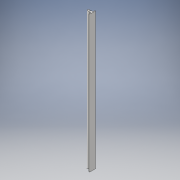
# Autodesk Inventor part: supportedRail_SBR12_750mm
Saved by Autodesk Inventor 2018 (Build 220112000, 112)
## iProperties
Created: 2020-03-10
Part Number: supportedRail_SBR12_750mm
Material: Generic
Document SubType Name: Modeling
Designer: natha
Density: 1 g/cm^3
Appearance: Default
Author: natha
Autodesk Inventor part; units mm, degrees
ref_plane "YZ Plane" through (0, 0, 0) normal (1, 0, 0) x (0, 1, 0)
ref_plane "XZ Plane" through (0, 0, 0) normal (0, 1, 0) x (-1, 0, 0)
ref_plane "XY Plane" through (0, 0, 0) normal (0, 0, 1) x (1, 0, 0)
sketch "Sketch1" plane through (0, 0, 0) normal (0, 1, 0) x (-1, 0, 0)
  line L0 (-22.5, -6) -> (-22.5, 6)
  line L1 (-10.5, -6) -> (-5.8469, -1.3469)
  line L2 (-10.5, -6) -> (-3.9195, -6) construction
  line L3 (-10.5, 6) -> (-5.8469, 1.3469)
  arc A0 (-5.8469, -1.3469) -> (-5.8469, 1.3469) centre (-0.0057, 0) ccw
  line L4 (-22.5, 16) -> (-22.5, -16)
  line L5 (-22.5, -16) -> (-18.5, -16)
  line L6 (-18.5, 16) -> (-22.5, 16)
  line L7 (-18.5, -16) -> (-18.5, -6)
  line L8 (-18.5, 16) -> (-18.5, 6)
  line L9 (-10.5, 6) -> (-18.5, 6)
  line L10 (-10.5, -6) -> (-18.5, -6)
  point P0 (0, 0)
  dimension "d2" = 12
  dimension "d3" = 45
  dimension "d4" = 12
  dimension "d6" = 5.9944
  dimension "d7" = 32
  dimension "d8" = 4
  dimension "d10" = 0
  constraints: 22 end point, 2 horizontal, 2 parallel, 2 point on circle, 1 centre point, 1 equal length, 1 perpendicular, 1 point on line, 1 vertical
  measures "d2" distance of L0.start L1.start
  measures "d3" angle of L2 L1
  measures "d4" distance of L0.end L3.start
  measures "d6" radius of A0
  measures "d7" distance of L4.start L4.end
  measures "d8" distance of L5.end L4.end
  measures "d10" distance between parallel lines of L0 L4
extrude "Extrusion1" add sketch "Sketch1" along normal blind 750
body "Solid1"
